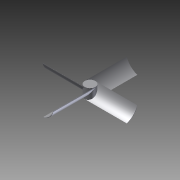
# Autodesk Inventor part: Fan
Saved by Autodesk Inventor 2012 (Build 160160000, 160)
## iProperties
Created: 2011-08-19
Part Number: Fan
Material: Default
Document SubType Name: Modeling
Designer: Minh Tran
Density: 1 g/cm^3
Author: Minh Tran
Autodesk Inventor part; units mm, degrees
sketch "Sketch1" plane through (0, 0, 0) normal (0, 0, 1) x (1, 0, 0)
  circle A0 centre (0, 0) radius 12.7
  dimension "d0" = 25.4
  constraints: 1 centre point, 1 coincident
  measures "d0" diameter of A0
extrude "Extrusion1" add sketch "Sketch1" along normal blind 25.4
ref_plane "Work Plane1" through (101.6, 0, 0) normal (1, 0, 0) x (0, 1, 0)
sketch "Sketch2" plane through (101.6, 0, 0) normal (1, 0, 0) x (0, 1, 0)
  arc A0 (-11.5079, 0) -> (12.6852, 24.1379) centre (-20.2903, 32.9957) ccw
  arc A1 (-12.7911, 0) -> (12.6852, 25.3834) centre (-25.5599, 38.2921) ccw
  line L0 (12.6852, 25.3834) -> (12.6852, 24.1379)
  line L1 (-12.7911, 0) -> (-11.5079, 0)
  point P0 (0, 0)
  constraints: 4 end point, 4 point on circle, 2 centre point, 1 perpendicular, 1 vertical
extrude "Extrusion2" add sketch "Sketch2" against normal blind 101.6
ref_plane "Work Plane2" through (0, -101.6, 0) normal (0, 1, 0) x (-1, 0, 0)
sketch "Sketch3" plane through (0, -101.6, 0) normal (0, 1, 0) x (-1, 0, 0)
  arc A0 (-12.7444, 23.4755) -> (10.8958, 0) centre (18.9573, 31.7588) ccw
  arc A1 (-12.7444, 25.3315) -> (12.6542, 0) centre (22.7301, 35.5012) ccw
  line L0 (-12.7444, 25.3315) -> (-12.7444, 23.4755)
  line L1 (12.6542, 0) -> (10.8958, 0)
  point P0 (0, 0)
  dimension "d7" = 32.766
  constraints: 6 point on circle, 4 end point, 2 centre point, 1 perpendicular, 1 vertical
  measures "d7" radius of A0
extrude "Extrusion3" add sketch "Sketch3" along normal blind 101.6
ref_plane "Work Plane3" through (-101.6, 0, 0) normal (1, 0, 0) x (0, 1, 0)
sketch "Sketch4" plane through (-101.6, 0, 0) normal (1, 0, 0) x (0, 1, 0)
  arc A0 (-12.7444, 23.4755) -> (10.8958, 0) centre (18.9573, 31.7588) ccw
  arc A1 (-12.7444, 25.3315) -> (12.6542, 0) centre (22.7301, 35.5012) ccw
  line L0 (-12.7444, 25.3315) -> (-12.7444, 23.4755)
  line L1 (12.6542, 0) -> (10.8958, 0)
  point P0 (0, 0)
  point P1 (0, 0)
  dimension "d11" = 32.766
  constraints: 6 point on circle, 4 end point, 2 centre point, 1 perpendicular, 1 vertical
  measures "d11" radius of A0
extrude "Extrusion4" add sketch "Sketch4" along normal blind 101.6
ref_plane "Work Plane4" through (0, 101.6, 0) normal (0, 1, 0) x (-1, 0, 0)
sketch "Sketch5" plane through (0, 101.6, 0) normal (0, 1, 0) x (-1, 0, 0)
  arc A0 (-11.5079, 0) -> (12.6852, 24.1379) centre (-20.2903, 32.9957) ccw
  arc A1 (-12.7911, 0) -> (12.6852, 25.3834) centre (-25.5599, 38.2921) ccw
  line L0 (12.6852, 25.3834) -> (12.6852, 24.1379)
  line L1 (-12.7911, 0) -> (-11.5079, 0)
  point P0 (0, 0)
  point P1 (0, 0)
  constraints: 4 end point, 4 point on circle, 2 centre point, 1 perpendicular, 1 vertical
extrude "Extrusion5" add sketch "Sketch5" against normal blind 101.6
body "Solid1"
